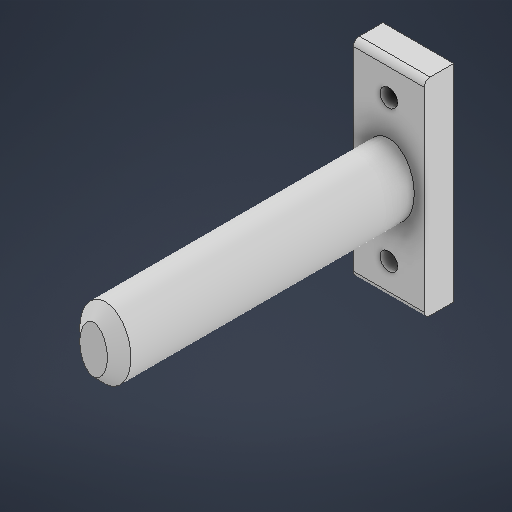
# Autodesk Inventor part: apoioM-mod
Saved by Autodesk Inventor 2026 (Build 300175050, 175E)
## iProperties
Created: 2025-06-17
Part Number: apoioM-mod
Material: Generic
Document SubType Name: Modeling
Designer: dcana
Density: 1 g/cm^3
Appearance: Default
Author: dcana
Autodesk Inventor part; units mm, degrees
ref_plane "YZ Plane" through (0, 0, 0) normal (1, 0, 0) x (0, 1, 0)
ref_plane "XZ Plane" through (0, 0, 0) normal (0, 1, 0) x (-1, 0, 0)
ref_plane "XY Plane" through (0, 0, 0) normal (0, 0, 1) x (1, 0, 0)
sketch "Sketch1" plane through (0, 0, 0) normal (0, 0, 1) x (1, 0, 0)
  circle A0 centre (-0.0139, -12) radius 1.5
  circle A1 centre (-0.0139, 12) radius 1.5
  line L0 (-6.0139, 17.5279) -> (5.9861, 17.5279)
  line L1 (5.9861, 17.5279) -> (5.9861, -17.4721)
  line L2 (5.9861, -17.4721) -> (-6.0139, -17.4721)
  line L3 (-6.0139, -17.4721) -> (-6.0139, 17.5279)
  line L4 (-0.0139, 12) -> (-0.0139, -12)
  line L5 (-0.0139, 12) -> (-0.0139, 5.686)
  ellipse E0 centre (-0.0442, 0.0279) end of major axis (-0.0442, 6.0549) minor radius 4.3359
  point P0 (0, 0)
  point P1 (-0.0139, -12)
  point P2 (-0.0139, 17.5279)
  dimension "d0" = 0
  dimension "d12" = 24
  dimension "d13" = 12
  constraints: 12 end point, 2 centre point, 2 parallel, 1 horizontal, 1 midpoint, 1 perpendicular, 1 point on line, 1 vertical, 2 other
  measures "d0" distance of point (-0.014, -12) L4.end
  measures "d12" distance of point (-0.014, -12) L4.start
  measures "d13" distance of L4.start point (0, 0)
extrude "Extrusion1" add sketch "Sketch1" along normal blind 5
sketch "Sketch2" plane through (0, 0, 5) normal (0, 0, 1) x (1, 0, 0)
  ellipse E0 centre (-0.0442, 0.0279) end of major axis (-0.0442, -5.9992) minor radius 4.3359 projected
  point P0 (0, 0)
  constraints: 1 other
extrude "Extrusion2" add sketch "Sketch2" along normal blind 50 and the other way blind 5
chamfer "Chamfer1" distance 2 angle 45 1 edges at (-0.0442, 6.0549, 55)
fillet "Fillet1" radius 1 1 edges at (-0.0139, 17.5279, 5)
fillet "Fillet2" radius 1 1 edges at (-0.0139, -17.4721, 5)
sketch "Sketch3" plane through (0, 0, 5) normal (0, 0, 1) x (1, 0, 0)
  point P0 (0, 0)
sketch "Sketch4" plane through (0, 0, 5) normal (0, 0, 1) x (1, 0, 0)
  point P0 (0, 0)
sketch "Sketch5" plane through (0, 0, 5) normal (0, 0, 1) x (1, 0, 0)
  point P0 (0, 0)
body "Solid1"
